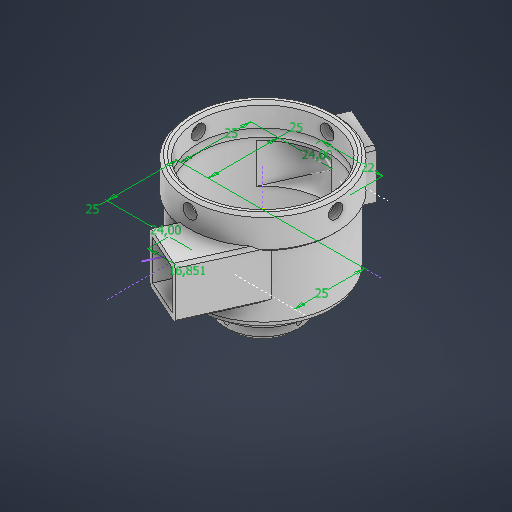
# Autodesk Inventor part: корпус ванночки
Saved by Autodesk Inventor 2026 (Build 300175000, 175)
## iProperties
Created: 2025-08-21
Part Number: корпус ванночки
Material: Типовые
Document SubType Name: Modeling
Designer: danil
Density: 1 g/cm^3
Appearance: По умолчанию
Author: danil
Autodesk Inventor part; units mm, degrees
ref_plane "YZ Plane" through (0, 0, 0) normal (1, 0, 0) x (0, 1, 0)
ref_plane "XZ Plane" through (0, 0, 0) normal (0, 1, 0) x (-1, 0, 0)
ref_plane "XY Plane" through (0, 0, 0) normal (0, 0, 1) x (1, 0, 0)
sketch "Эскиз5" plane through (0, 0, 0) normal (1, 0, 0) x (0, 1, 0)
  line L0 (7, -23) -> (1.6898, -16.3063)
  line L1 (1.6898, -16.3063) -> (0, -10)
  line L2 (0, -10) -> (-8, -10)
  line L3 (-1.294, -13) -> (-0.1589, -17.2365)
  line L4 (-0.1589, -17.2365) -> (6, -25)
  line L5 (6, -25) -> (36, -25)
  line L6 (-1.294, -13) -> (-8, -13)
  line L7 (7, -23) -> (36, -23)
  line L8 (36, -23) -> (36, -25)
  line L9 (-8, -10) -> (-8, -13)
  line L10 (0, 0) -> (0, -60) construction
  line L11 (0, 0) -> (9.798, 0)
  point P0 (36, -24)
  dimension "d12" = 2
  dimension "d13" = 30
  dimension "d14" = 36
  dimension "d15" = 3
  dimension "d17" = 29
  dimension "d18" = 23
  dimension "d20" = 10
  dimension "d23" = 60
  dimension "d24" = 15
  dimension "d26" = 38.425
  dimension "d87" = 8
  constraints: 24 end point, 3 parallel, 2 horizontal, 2 perpendicular, 1 midpoint, 1 point on line, 1 vertical, 1 other
  measures "d12" distance of L7.end L5.end
  measures "d13" distance of L4.end L5.end
  measures "d14" horizontal distance of L10.start point (36, -24)
  measures "d15" distance of L2.end L6.end
  measures "d17" distance of L0.start L7.end
  measures "d18" vertical distance of L10.start L0.start
  measures "d20" distance of L10.start L1.end
  measures "d23" distance of L10.start L10.end
  measures "d24" angle of L10 L1
  measures "d26" angle of L10 L4
  measures "d87" distance of L1.end L2.end
revolve "Вращение1" add sketch "Эскиз5" angle 360 about axis through (0, 0, 0) along (0, 1, 0)
ref_plane "РабПлоскость2" through (0, 24, 0) normal (0, 1, 0) x (1, 0, 0)
ref_plane "РабПлоскость1" through (0, 36, 0) normal (0, 1, 0) x (1, 0, 0)
sketch "Эскиз6" plane through (0, 24, 0) normal (0, 1, 0) x (1, 0, 0)
  line L0 (-8.4256, -21.2487) -> (8.4256, -28.7513)
  line L1 (0, 0) -> (0, -55.745) construction
  line L2 (0, 0) -> (42.4621, 0) construction
  line L3 (40.8556, -25) -> (-23.1238, -25) construction
  line L4 (0, -25) -> (-5.5208, -37.3998)
  dimension "d29" = 25
  dimension "d30" = 25
  dimension "d31" = 24
  dimension "d35" = 16.8512
  constraints: 10 end point, 2 horizontal, 1 midpoint, 1 perpendicular, 1 point on line, 1 vertical
  measures "d29" distance from line of L3 point (0, 0)
  measures "d30" distance of L4.start point (0, 0)
  measures "d31" angle of L3 L0
  measures "d35" horizontal distance of L0.start L0.end
ref_plane "РабПлоскость4" through (-8.4256, 24, 21.2487) normal (-0.4067366, 0, 0.9135455) x (0.9135455, 0, 0.4067366)
sketch "Эскиз9" plane through (-8.4256, 24, 21.2487) normal (-0.4067366, 0, 0.9135455) x (0.9135455, 0, 0.4067366)
  line L0 (7.0546, 5) -> (21.0546, 5)
  line L1 (21.0546, 5) -> (21.0546, -9)
  line L2 (21.0546, -9) -> (7.0546, -9)
  line L3 (7.0546, -9) -> (7.0546, 5)
  line L4 (24.0546, 12) -> (-25.9454, 12) projected
  line L5 (24.0546, -18) -> (-25.9454, -18) projected
  point P0 (-0.9454, -24)
  point P1 (14.0546, 5)
  dimension "d38" = 14
  dimension "d39" = 14
  dimension "d41" = 22
  dimension "d54" = 9
  constraints: 8 end point, 2 parallel, 1 horizontal, 1 midpoint, 1 perpendicular
  measures "d38" distance of L0.start L0.end
  measures "d39" distance of L0.end L1.end
  measures "d41" horizontal distance of point (-0.945, -24) L0.end
  measures "d54" distance from line of L5 L1.end
extrude "Выдавливание4" cut sketch "Эскиз9" along normal blind 12 and the other way blind 22
sketch "Эскиз10" plane through (-8.4256, 24, 21.2487) normal (-0.4067366, 0, 0.9135455) x (0.9135455, 0, 0.4067366)
  line L0 (5.0546, 7) -> (23.0546, 7)
  line L1 (23.0546, 7) -> (23.0546, -11)
  line L2 (23.0546, -11) -> (5.0546, -11)
  line L3 (5.0546, -11) -> (5.0546, 7)
  line L4 (24.0546, 12) -> (-25.9454, 12) projected
  line L5 (7.0546, 5) -> (21.0546, 5) projected
  line L6 (7.0546, 5) -> (21.0546, 5)
  line L7 (21.0546, 5) -> (21.0546, -9)
  line L8 (21.0546, -9) -> (7.0546, -9)
  line L9 (7.0546, -9) -> (7.0546, 5)
  line L10 (24.0546, -18) -> (-25.9454, -18) projected
  point P0 (-0.9454, -24)
  dimension "d46" = 18
  dimension "d47" = 18
  dimension "d49" = 24
  dimension "d56" = 7
  constraints: 16 end point, 4 parallel, 2 horizontal, 2 perpendicular
  measures "d46" distance of L0.start L0.end
  measures "d47" distance of L0.end L1.end
  measures "d49" horizontal distance of point (-0.945, -24) L0.end
  measures "d56" vertical distance of L10.start L1.end
extrude "Выдавливание5" add sketch "Эскиз10" along normal blind 10 and the other way blind 22
sketch "Эскиз11" plane through (0, 24, 0) normal (0, 1, 0) x (1, 0, 0)
  line L0 (11, 20.1025) -> (-11, 29.8975)
  line L1 (19.4489, 25) -> (-19.4489, 25) construction
  line L2 (0, 25) -> (-2.3969, 19.6164) construction
  point P0 (0, 0)
  dimension "d57" = 25
  dimension "d59" = 22
  dimension "d60" = 25
  dimension "d61" = 24
  constraints: 6 end point, 3 midpoint, 1 horizontal, 1 perpendicular, 1 point on line
  measures "d57" distance of point (0, 0) L2.start
  measures "d59" horizontal distance of L0.start L0.end
  measures "d60" distance of point (0, 0) L2.start
  measures "d61" angle of L0 L1
ref_plane "РабПлоскость5" through (11, 24, -20.1025) normal (0.4067366, 0, -0.9135455) x (-0.9135455, 0, -0.4067366)
sketch "Эскиз12" plane through (11, 24, -20.1025) normal (0.4067366, 0, -0.9135455) x (-0.9135455, 0, -0.4067366)
  line L0 (9.8726, 5) -> (23.8726, 5)
  line L1 (23.8726, 5) -> (23.8726, -9)
  line L2 (23.8726, -9) -> (9.8726, -9)
  line L3 (9.8726, -9) -> (9.8726, 5)
  line L4 (26.8726, -18) -> (-23.1274, -18) projected
  point P0 (1.8726, -24)
  dimension "d63" = 14
  dimension "d64" = 14
  dimension "d65" = 9
  dimension "d66" = 22
  constraints: 8 end point, 2 parallel, 1 horizontal, 1 perpendicular
  measures "d63" distance of L0.start L0.end
  measures "d64" distance of L0.end L1.end
  measures "d65" distance from line of L4 L1.end
  measures "d66" horizontal distance of point (1.873, -24) L1.end
extrude "Выдавливание6" cut sketch "Эскиз12" along normal blind 12 and the other way blind 22
sketch "Эскиз13" plane through (11, 24, -20.1025) normal (0.4067366, 0, -0.9135455) x (-0.9135455, 0, -0.4067366)
  line L0 (23.8726, 5) -> (9.8726, 5) projected
  line L1 (23.8726, -9) -> (9.8726, -9) projected
  line L2 (9.8726, 5) -> (23.8726, 5)
  line L3 (23.8726, 5) -> (23.8726, -9)
  line L4 (23.8726, -9) -> (9.8726, -9)
  line L5 (9.8726, -9) -> (9.8726, 5)
  line L6 (7.8726, 7) -> (25.8726, 7)
  line L7 (25.8726, 7) -> (25.8726, -11)
  line L8 (25.8726, -11) -> (7.8726, -11)
  line L9 (7.8726, -11) -> (7.8726, 7)
  line L10 (26.8726, -18) -> (-23.1274, -18) projected
  point P0 (1.8726, -24)
  point P1 (9.8726, -9)
  dimension "d71" = 18
  dimension "d72" = 18
  dimension "d74" = 7
  dimension "d75" = 24
  constraints: 16 end point, 4 parallel, 2 horizontal, 2 perpendicular
  measures "d71" distance of L6.start L6.end
  measures "d72" distance of L6.end L7.end
  measures "d74" distance from line of L10 L7.end
  measures "d75" horizontal distance of point (1.873, -24) L7.end
extrude "Выдавливание7" add sketch "Эскиз13" along normal blind 10 and the other way blind 22
ref_plane "РабПлоскость6" through (0, 36, 0) normal (0, 1, 0) x (1, 0, 0)
sketch "Эскиз14" plane through (0, 36, 0) normal (0, 1, 0) x (1, 0, 0)
  circle A0 centre (0, 0) radius 23
  dimension "d81" = 46
  constraints: 1 centre point, 1 coincident
  measures "d81" diameter of A0
extrude "Выдавливание8" cut sketch "Эскиз14" against normal blind 24
chamfer "Фаска1" distance 2 angle 45 1 edges at (0, -8, 13)
sketch "Эскиз16" plane through (0, 36, 0) normal (0, 1, 0) x (1, 0, 0)
  circle A0 centre (0, 0) radius 23
  circle A1 centre (0, 0) radius 25
  constraints: 2 centre point, 2 coincident
extrude "Выдавливание9" add sketch "Эскиз16" along normal blind 5
sketch "Эскиз17" plane through (0, 41, 0) normal (0, 1, 0) x (1, 0, 0)
  circle A0 centre (0, 0) radius 25
  circle A1 centre (0, 0) radius 26
  dimension "d90" = 52
  dimension "d91" = 50
  constraints: 2 centre point, 2 coincident
  measures "d90" diameter of A1
  measures "d91" diameter of A0
extrude "Выдавливание10" add sketch "Эскиз17" against normal blind 12
sketch "Эскиз18" plane through (0, 0, 0) normal (1, 0, 0) x (0, 1, 0)
  circle A0 centre (36.5, 0) radius 2.5
  line L0 (41, 23) -> (41, -23) projected
  point P0 (0, 0)
  dimension "d94" = 0
  dimension "d96" = 5
  dimension "d99" = 4.5
  constraints: 1 centre point
  measures "d94" vertical distance of point (0, 0) A0.centre
  measures "d96" diameter of A0
  measures "d99" distance from line of A0.centre L0
extrude "Выдавливание11" cut sketch "Эскиз18" along normal mid plane 60
sketch "Эскиз19" plane through (0, 0, 0) normal (0, 0, 1) x (1, 0, 0)
  circle A0 centre (0, 36.5) radius 2.5
  line L0 (-23, 41) -> (23, 41) projected
  point P0 (0, 0)
  dimension "d100" = 0
  dimension "d101" = 4.5
  dimension "d102" = 5
  constraints: 1 centre point
  measures "d100" horizontal distance of point (0, 0) A0.centre
  measures "d101" distance from line of L0 A0.centre
  measures "d102" diameter of A0
extrude "Выдавливание12" cut sketch "Эскиз19" along normal mid plane 60
sketch "Эскиз20" plane through (0, 0, 0) normal (1, 0, 0) x (0, 1, 0)
  circle A0 centre (31.5, -22.5) radius 1.5
  line L0 (41, 23) -> (41, -23) projected
  point P0 (0, 0)
  dimension "d105" = 9.5
  dimension "d107" = 3
  dimension "d108" = 22.5
  constraints: 1 centre point
  measures "d105" distance from line of L0 A0.centre
  measures "d107" diameter of A0
  measures "d108" vertical distance of point (0, 0) A0.centre
sketch "Эскиз21" plane through (0, 0, 0) normal (1, 0, 0) x (0, 1, 0)
  line L0 (8.5737, 0) -> (21.9208, 0) construction
  line L1 (19.2198, 0) -> (37.6208, 0) construction
  point P0 (0, 0)
  constraints: 4 end point, 2 point on line, 1 horizontal
revolve "Вращение2" cut sketch "Эскиз20" angle 360 about axis through (0, 19.2198, 0) along (0, 1, 0)
sketch "Эскиз22" plane through (0, 0, 0) normal (1, 0, 0) x (0, 1, 0)
  circle A0 centre (-4, 0) radius 1
  line L0 (-8, -11) -> (-8, 11) projected
  point P0 (0, 0)
  point P1 (-8, 0)
  dimension "d110" = 4
  dimension "d111" = 0
  dimension "d112" = 2
  constraints: 1 centre point, 1 midpoint
  measures "d110" distance from line of L0 A0.centre
  measures "d111" vertical distance of point (-8, 0) A0.centre
  measures "d112" diameter of A0
extrude "Выдавливание13" cut sketch "Эскиз22" along normal mid plane 30
sketch "Эскиз23" plane through (0, 0, 0) normal (0, 0, 1) x (1, 0, 0)
  circle A0 centre (0, -4) radius 1
  line L0 (11, -8) -> (-11, -8) projected
  point P0 (0, 0)
  point P1 (0, -8)
  dimension "d115" = 4
  dimension "d116" = 0
  dimension "d117" = 2
  constraints: 1 centre point, 1 midpoint
  measures "d115" distance from line of L0 A0.centre
  measures "d116" horizontal distance of point (0, -8) A0.centre
  measures "d117" diameter of A0
extrude "Выдавливание14" cut sketch "Эскиз23" along normal mid plane 30
thread "Резьба1" size "M5x0.8" class "6H" standard "ANSI Metric M Profile" full length
thread "Резьба2" size "M5x0.8" class "6H" standard "ANSI Metric M Profile" full length
thread "Резьба3" size "M5x0.8" class "6H" standard "ANSI Metric M Profile" full length
thread "Резьба4" size "M5x0.8" class "6H" standard "ANSI Metric M Profile" full length
thread "Резьба5" size "M2x0.4" class "6H" standard "ANSI Metric M Profile" full length
thread "Резьба6" size "M2x0.4" class "6H" standard "ANSI Metric M Profile" full length
thread "Резьба7" size "M2x0.4" class "6H" standard "ANSI Metric M Profile" full length
thread "Резьба8" size "M2x0.4" class "6H" standard "ANSI Metric M Profile" full length
chamfer "Фаска2" distance 1 angle 45 13 edges at (23.8778, 29, 10.2883) (20.0127, 29, -16.5979) (-24.9471, 29, 7.324) (13.2131, 31, 29.3292) (-6.3419, 31, 28.9958) (-6.1327, 13, 28.5258) (13.8232, 13, 27.9589) (-13.2131, 31, -29.3292) (6.3419, 31, -28.9958) (6.1327, 13, -28.5258) (-13.8232, 13, -27.9589) (0, 6, 25) (-26, 41, 0)
chamfer "Фаска3" distance 1 angle 45 1 edges at (-23, 41, 0)
